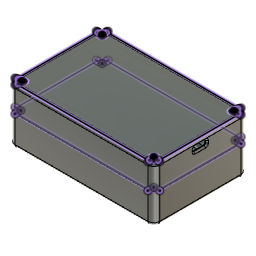
Servotester Case (Autodesk Fusion 360 design; units mm, degrees)
Autodesk Fusion 360 part; units mm, degrees
sketch "Skizze1" plane through (0, 0, 0) normal (0, 0, 1) x (1, 0, 0)
  line L0 (6.5, 58) -> (88.5, 58) construction
  line L1 (88.5, 58) -> (88.5, 21.5) construction
  line L2 (88.5, 21.5) -> (6.5, 21.5) construction
  line L3 (6.5, 21.5) -> (6.5, 58) construction
  line L4 (11.5, 52.5) -> (83.5, 52.5)
  line L5 (83.5, 52.5) -> (83.5, 27.5)
  line L6 (83.5, 27.5) -> (11.5, 27.5)
  line L7 (11.5, 27.5) -> (11.5, 52.5)
  circle A0 centre (10, 55.5) radius 1.5
  line L8 (35, 21.4) -> (61.3, 21.4) construction
  line L9 (61.3, 21.4) -> (61.3, 2.2) construction
  line L10 (61.3, 2.2) -> (35, 2.2) construction
  line L11 (35, 2.2) -> (35, 21.4) construction
  line L12 (8.4, 19.5) -> (19, 19.5) construction
  line L13 (19, 19.5) -> (19, 4.5) construction
  line L14 (19, 4.5) -> (8.4, 4.5) construction
  line L15 (8.4, 4.5) -> (8.4, 19.5) construction
  line L16 (72.4, 14.15) -> (80.4, 14.15)
  line L17 (80.4, 14.15) -> (80.4, 8.45)
  line L18 (80.4, 8.45) -> (72.4, 8.45)
  line L19 (72.4, 8.45) -> (72.4, 14.15)
  line L20 (9.25, 19.2) -> (18.15, 19.2)
  line L21 (18.15, 19.2) -> (18.15, 4.8)
  line L22 (18.15, 4.8) -> (9.25, 4.8)
  line L23 (9.25, 4.8) -> (9.25, 19.2)
  circle A1 centre (50.6, 10.1) radius 3.7
  line L24 (66.3, 21.4) -> (86.5, 21.4) construction
  line L25 (86.5, 21.4) -> (86.5, 1.2) construction
  line L26 (86.5, 1.2) -> (66.3, 1.2) construction
  line L27 (66.3, 1.2) -> (66.3, 21.4) construction
  circle A2 centre (71.32, 17.65) radius 1.5
  circle A3 centre (81.48, 17.65) radius 1.5
  circle A4 centre (71.32, 4.95) radius 1.5
  circle A5 centre (81.48, 4.95) radius 1.5
  circle A6 centre (85, 55.5) radius 1.5
  circle A7 centre (10, 24.5) radius 1.5
  circle A8 centre (85, 24.5) radius 1.5
  circle A9 centre (10, 55.5) radius 3
  circle A10 centre (85, 55.5) radius 3
  circle A11 centre (10, 24.5) radius 3
  circle A12 centre (85, 24.5) radius 3
  circle A13 centre (71.32, 17.65) radius 3
  circle A14 centre (81.48, 17.65) radius 3
  circle A15 centre (71.32, 4.95) radius 3
  circle A16 centre (81.48, 4.95) radius 3
  line L28 (2.5, 60) -> (92.5, 60)
  line L29 (95, 57.5) -> (95, 2.5)
  line L30 (92.5, 0) -> (2.5, 0)
  line L31 (0, 2.5) -> (0, 57.5)
  arc A17 (2.5, 60) -> (0, 57.5) centre (2.5, 57.5) ccw
  arc A18 (95, 57.5) -> (92.5, 60) centre (92.5, 57.5) ccw
  arc A19 (92.5, 0) -> (95, 2.5) centre (92.5, 2.5) ccw
  arc A20 (0, 2.5) -> (2.5, 0) centre (2.5, 2.5) ccw
  arc A21 (96.5, 57.5) -> (92.5, 61.5) centre (92.5, 57.5) ccw
  line L32 (2.5, 61.5) -> (92.5, 61.5)
  arc A22 (2.5, 61.5) -> (-1.5, 57.5) centre (2.5, 57.5) ccw
  line L33 (-1.5, 2.5) -> (-1.5, 57.5)
  arc A23 (-1.5, 2.5) -> (2.5, -1.5) centre (2.5, 2.5) ccw
  line L34 (92.5, -1.5) -> (2.5, -1.5)
  arc A24 (92.5, -1.5) -> (96.5, 2.5) centre (92.5, 2.5) ccw
  line L35 (96.5, 57.5) -> (96.5, 2.5)
  circle A25 centre (3, 57) radius 3
  circle A26 centre (92, 57) radius 3
  circle A27 centre (92, 3) radius 3
  circle A28 centre (3, 3) radius 3
  circle A29 centre (3, 57) radius 1.5
  circle A30 centre (92, 57) radius 1.5
  circle A31 centre (92, 3) radius 1.5
  circle A32 centre (3, 3) radius 1.5
  point P0 (0, 60)
  point P1 (95, 60)
  dimension "d3" = 82
  dimension "d4" = 36.5
  dimension "d5" = 72
  dimension "d6" = 25
  dimension "d15" = 3
  dimension "d16" = 2.5
  dimension "d20" = 26.3
  dimension "d21" = 19.2
  dimension "d22" = 10.6
  dimension "d23" = 15
  dimension "d24" = 8
  dimension "d25" = 5.7
  dimension "d26" = 8.9
  dimension "d27" = 14.4
  dimension "d28" = 0.85
  dimension "d29" = 0.3
  dimension "d30" = 7.4
  dimension "d31" = 7.9
  dimension "d32" = 10.7
  dimension "d35" = 16
  dimension "d39" = 20.2
  dimension "d40" = 20.2
  dimension "d43" = 6.1
  dimension "d44" = 7.25
  dimension "d45" = 3
  dimension "d49" = 10.16
  dimension "d50" = -12.7
  dimension "d51" = 5.02
  dimension "d52" = 3.75
  dimension "d59" = 75
  dimension "d60" = -31
  dimension "d61" = 5
  dimension "d62" = 0.1
  dimension "d63" = 0.1
  dimension "d64" = 2
  dimension "d65" = 3.5
  dimension "d66" = 2
  dimension "d67" = 6
  dimension "d68" = 5.5
  dimension "d69" = 5
  dimension "d70" = 6
  dimension "d71" = 2
  dimension "d72" = 6.5
  dimension "d74" = 60
  dimension "d75" = 2.5
  dimension "d76" = -1.5
  dimension "d83" = 6
  dimension "d84" = 6.5
  dimension "d85" = 6
  dimension "d86" = 6
  dimension "d87" = 6
  dimension "d88" = 3
  dimension "d89" = 3
  dimension "d90" = 3
  dimension "d91" = 3
  constraint horizontal L0
  constraint vertical L1
  constraint horizontal L2
  constraint vertical L3
  constraint horizontal L4
  constraint vertical L5
  constraint horizontal L6
  constraint vertical L7
  constraint horizontal L8
  constraint vertical L9
  constraint horizontal L10
  constraint vertical L11
  constraint horizontal L12
  constraint vertical L13
  constraint horizontal L14
  constraint vertical L15
  constraint horizontal L16
  constraint vertical L17
  constraint horizontal L18
  constraint vertical L19
  constraint horizontal L20
  constraint vertical L21
  constraint horizontal L22
  constraint vertical L23
  constraint horizontal L24
  constraint vertical L25
  constraint horizontal L26
  constraint vertical L27
  constraint concentric A0 A9
  constraint concentric A2 A13
  constraint horizontal L28
  constraint vertical L29
  constraint horizontal L30
  constraint vertical L31
  constraint coincident P0 L31
  constraint coincident P0 L28
  constraint tangent L31 A17
  constraint tangent L28 A17
  constraint coincident P1 L28
  constraint coincident P1 L29
  constraint tangent L28 A18
  constraint tangent L29 A18
  constraint equal A17 A18
  constraint tangent L29 A19
  constraint tangent L30 A19
  constraint equal A17 A19
  constraint coincident origin L30
  constraint coincident origin L31
  constraint tangent L30 A20
  constraint tangent L31 A20
  constraint equal A17 A20
  constraint tangent L28 A25
  constraint tangent L31 A25
  constraint tangent L28 A26
  constraint tangent L29 A26
  constraint tangent L30 A28
  constraint tangent L31 A28
  constraint tangent L30 A27
  constraint tangent L29 A27
  constraint concentric A25 A29
  constraint concentric A26 A30
  constraint concentric A27 A31
  constraint concentric A28 A32
  measures "d3" distance of L0.start L0.end
  measures "d4" distance of L0.start L2.end
  measures "d5" distance of L4.start L4.end
  measures "d6" distance of L4.start L6.end
  measures "d15" diameter of A0
  measures "d16" distance of L0 A0.centre
  measures "d20" distance of L8.start L8.end
  measures "d21" distance of L8.start L10.end
  measures "d22" distance of L12.start L12.end
  measures "d23" distance of L12.start L14.end
  measures "d24" distance of L16.start L16.end
  measures "d25" distance of L16.start L18.end
  measures "d26" distance of L20.start L20.end
  measures "d27" distance of L20.start L22.end
  measures "d28" distance of L15 L23
  measures "d29" distance of L12 L20
  measures "d30" diameter of A1
  measures "d31" distance of L10 A1.centre
  measures "d32" distance of L9 A1.centre
  measures "d35" distance of L11 L13
  measures "d39" distance of L24.start L24.end
  measures "d40" distance of L24.start L26.end
  measures "d43" distance of L19 L27
  measures "d44" distance of L18 L26
  measures "d45" diameter of A2
  measures "d51" distance of L27 A2.centre
  measures "d52" distance of L24 A2.centre
  measures "d61" distance of L9 L27
  measures "d62" distance of L2 L8
  measures "d63" distance of L2 L24
  measures "d64" distance of L2 L12
  measures "d65" distance of L3 A0.centre
  measures "d66" distance of L1 L25
  measures "d67" diameter of A9
  measures "d68" distance of L0 L4
  measures "d69" distance of L3 L7
  measures "d70" diameter of A13
  measures "d71" distance of L0 L28
  measures "d72" distance of L1 L29
  measures "d74" distance of P0 origin
  measures "d75" radius of A17
  measures "d83" diameter of A25
  measures "d84" distance of L3 L31
  measures "d85" diameter of A26
  measures "d86" diameter of A27
  measures "d87" diameter of A28
  measures "d88" diameter of A29
  measures "d89" diameter of A30
  measures "d90" diameter of A31
  measures "d91" diameter of A32
extrude "Extrusion1" add sketch "Skizze1" along normal blind 1.5 contours A0 | A2 | A3 | A4 | A5 | A6 | A7 | A8 | A9 | A10 | A11 | A12 | A13 | A14 | A15 | A16 | L28 L31 A17 A25 | L28 L29 L30 L31 A25 A26 A27 A28 | A25 | L28 L29 A18 A26 | A26 | L30 L31 A20 A28 | A28 | A27 | L29 L30 A19 A27 | A29 | A30 | A31 | A32 makes body 1
extrude "Extrusion2" add sketch "Skizze1" along normal blind 6 contours A9 | A10 | A11 | A12 bodies 1
extrude "Extrusion12" add sketch "Skizze1" along normal blind 4.4 contours A13 | A14 | A15 | A16 bodies 1
extrude "Extrusion4" add sketch "Skizze1" along normal blind 15 contours L28 L31 A17 A25 | A25 | L28 L29 A18 A26 | A26 | L30 L31 A20 A28 | A28 | A27 | L29 L30 A19 A27 bodies 1
extrude "Extrusion3" add sketch "Skizze1" along normal blind 20 contours A21 L32 A22 L33 A23 L34 A24 L35 bodies 1
fillet "Abrundung1" radius 2 8 edges at (-0.3284, -0.3284, 0) (47.5, -1.5, 0) (95.3284, -0.3284, 0) (96.5, 30, 0) (95.3284, 60.3284, 0) (47.5, 61.5, 0) (-0.3284, 60.3284, 0) (-1.5, 30, 0) on bodies 1
chamfer "Fase1" distance 0.8 angle 45 8 edges at (72.4, 11.3, 0) (80.4, 11.3, 0) (76.4, 8.45, 0) (76.4, 14.15, 0) (11.5, 40, 0) (47.5, 52.5, 0) (83.5, 40, 0) (47.5, 27.5, 0) on bodies 1
fillet "Abrundung2" radius 2 8 edges at (47.5, 0, 1.5) (95, 30, 1.5) (89.8787, 5.1213, 1.5) (5.1213, 5.1213, 1.5) (0, 30, 1.5) (5.1213, 54.8787, 1.5) (47.5, 60, 1.5) (89.8787, 54.8787, 1.5) on bodies 1
fillet "Abrundung5" radius 1 4 edges at (82.203, 25.5848, 1.5) (78.683, 18.7348, 1.5) (68.523, 18.7348, 1.5) (7.203, 25.5848, 1.5) on bodies 1
fillet "Abrundung6" radius 0.5 4 edges at (81.48, 1.95, 1.5006) (81.48, 7.95, 1.5) (71.32, 1.95, 1.5006) (71.32, 7.95, 1.5) on bodies 1
sketch "Skizze2" plane through (0, 0, 20) normal (0, 0, 1) x (-1, 0, 0)
  arc A0 (-2.5, -60) -> (0, -57.5) centre (-2.5, -57.5) ccw
  line L0 (-2.5, -60) -> (-92.5, -60)
  arc A1 (-95, -57.5) -> (-92.5, -60) centre (-92.5, -57.5) ccw
  line L1 (-95, -57.5) -> (-95, -2.5)
  arc A2 (-92.5, 0) -> (-95, -2.5) centre (-92.5, -2.5) ccw
  line L2 (-92.5, 0) -> (-2.5, 0)
  arc A3 (0, -2.5) -> (-2.5, 0) centre (-2.5, -2.5) ccw
  line L3 (0, -2.5) -> (0, -57.5)
  arc A4 (-2.5, -61.5) -> (1.5, -57.5) centre (-2.5, -57.5) ccw
  line L4 (1.5, -57.5) -> (1.5, -2.5)
  arc A5 (1.5, -2.5) -> (-2.5, 1.5) centre (-2.5, -2.5) ccw
  line L5 (-2.5, 1.5) -> (-92.5, 1.5)
  arc A6 (-92.5, 1.5) -> (-96.5, -2.5) centre (-92.5, -2.5) ccw
  line L6 (-96.5, -2.5) -> (-96.5, -57.5)
  arc A7 (-96.5, -57.5) -> (-92.5, -61.5) centre (-92.5, -57.5) ccw
  line L7 (-92.5, -61.5) -> (-2.5, -61.5)
  line L8 (-95.7, -2.5) -> (-95.7, -57.5)
  arc A8 (-95.7, -57.5) -> (-92.5, -60.7) centre (-92.5, -57.5) ccw
  line L9 (-92.5, -60.7) -> (-2.5, -60.7)
  arc A9 (-2.5, -60.7) -> (0.7, -57.5) centre (-2.5, -57.5) ccw
  line L10 (0.7, -57.5) -> (0.7, -2.5)
  arc A10 (0.7, -2.5) -> (-2.5, 0.7) centre (-2.5, -2.5) ccw
  line L11 (-2.5, 0.7) -> (-92.5, 0.7)
  arc A11 (-92.5, 0.7) -> (-95.7, -2.5) centre (-92.5, -2.5) ccw
  dimension "d99" = -0.8
extrude "Extrusion5" cut sketch "Skizze2" against normal blind 1.5 contours L8 A8 L9 A9 L10 A10 L11 A11 bodies 1
ref_plane "Arbeitsebene1" through (47.5, 30, 37) normal (0, 0, -1) x (-1, 0, 0)
sketch "Skizze3" plane through (48.2, 30, 37) normal (0, 0, -1) x (1, 0, 0)
  line L0 (47.5, -27.5) -> (47.5, 27.5)
  arc A0 (47.5, 27.5) -> (44.3, 30.7) centre (44.3, 27.5) ccw
  line L1 (44.3, 30.7) -> (-45.7, 30.7)
  arc A1 (-45.7, 30.7) -> (-48.9, 27.5) centre (-45.7, 27.5) ccw
  line L2 (-48.9, 27.5) -> (-48.9, -27.5)
  arc A2 (-48.9, -27.5) -> (-45.7, -30.7) centre (-45.7, -27.5) ccw
  line L3 (-45.7, -30.7) -> (44.3, -30.7)
  arc A3 (44.3, -30.7) -> (47.5, -27.5) centre (44.3, -27.5) ccw
  arc A4 (-49.7, -27.5) -> (-45.7, -31.5) centre (-45.7, -27.5) ccw
  line L4 (-49.7, -27.5) -> (-49.7, 27.5)
  arc A5 (-45.7, 31.5) -> (-49.7, 27.5) centre (-45.7, 27.5) ccw
  line L5 (-45.7, 31.5) -> (44.3, 31.5)
  arc A6 (48.3, 27.5) -> (44.3, 31.5) centre (44.3, 27.5) ccw
  line L6 (48.3, 27.5) -> (48.3, -27.5)
  arc A7 (44.3, -31.5) -> (48.3, -27.5) centre (44.3, -27.5) ccw
  line L7 (44.3, -31.5) -> (-45.7, -31.5)
  arc A8 (46.8, 27.5) -> (44.3, 30) centre (44.3, 27.5) ccw
  line L8 (44.3, 30) -> (-45.7, 30)
  arc A9 (-45.7, 30) -> (-48.2, 27.5) centre (-45.7, 27.5) ccw
  line L9 (-48.2, 27.5) -> (-48.2, -27.5)
  arc A10 (-48.2, -27.5) -> (-45.7, -30) centre (-45.7, -27.5) ccw
  line L10 (-45.7, -30) -> (44.3, -30)
  arc A11 (44.3, -30) -> (46.8, -27.5) centre (44.3, -27.5) ccw
  line L11 (46.8, -27.5) -> (46.8, 27.5)
  arc A12 (47.5, 27.5) -> (44.3, 30.7) centre (44.3, 27.5) ccw
  line L12 (47.5, 27.5) -> (47.5, -27.5)
  arc A13 (44.3, -30.7) -> (47.5, -27.5) centre (44.3, -27.5) ccw
  line L13 (44.3, -30.7) -> (-45.7, -30.7)
  arc A14 (-48.9, -27.5) -> (-45.7, -30.7) centre (-45.7, -27.5) ccw
  line L14 (-48.9, -27.5) -> (-48.9, 27.5)
  arc A15 (-45.7, 30.7) -> (-48.9, 27.5) centre (-45.7, 27.5) ccw
  line L15 (-45.7, 30.7) -> (44.3, 30.7)
  circle A16 centre (43.8, 27) radius 1.5
  arc A17 (46.8, 27.5) -> (44.3, 30) centre (44.3, 27.5) ccw
  line L16 (46.8, 27.5) -> (46.8, 27)
  arc A18 (43.8, 30) -> (46.8, 27) centre (43.8, 27) ccw
  line L17 (43.8, 30) -> (44.3, 30)
  circle A19 centre (-45.2, 27) radius 1.5
  arc A20 (-45.7, 30) -> (-48.2, 27.5) centre (-45.7, 27.5) ccw
  line L18 (-45.7, 30) -> (-45.2, 30)
  arc A21 (-48.2, 27) -> (-45.2, 30) centre (-45.2, 27) ccw
  line L19 (-48.2, 27) -> (-48.2, 27.5)
  circle A22 centre (-45.2, -27) radius 1.5
  arc A23 (-48.2, -27.5) -> (-45.7, -30) centre (-45.7, -27.5) ccw
  line L20 (-48.2, -27.5) -> (-48.2, -27)
  arc A24 (-45.2, -30) -> (-48.2, -27) centre (-45.2, -27) ccw
  line L21 (-45.2, -30) -> (-45.7, -30)
  circle A25 centre (43.8, -27) radius 1.5
  arc A26 (44.3, -30) -> (46.8, -27.5) centre (44.3, -27.5) ccw
  line L22 (44.3, -30) -> (43.8, -30)
  arc A27 (46.8, -27) -> (43.8, -30) centre (43.8, -27) ccw
  line L23 (46.8, -27) -> (46.8, -27.5)
  circle A28 centre (43.8, 27) radius 1.2
  circle A29 centre (43.8, 27) radius 2.1
  circle A30 centre (-45.2, 27) radius 1.2
  circle A31 centre (-45.2, 27) radius 2.1
  circle A32 centre (43.8, -27) radius 1.2
  circle A33 centre (43.8, -27) radius 2.1
  circle A34 centre (-45.2, -27) radius 1.2
  circle A35 centre (-45.2, -27) radius 2.1
  line L24 (-45.7, -30.5) -> (44.3, -30.5)
  arc A36 (44.3, -30.5) -> (47.3, -27.5) centre (44.3, -27.5) ccw
  line L25 (47.3, -27.5) -> (47.3, 27.5)
  arc A37 (47.3, 27.5) -> (44.3, 30.5) centre (44.3, 27.5) ccw
  line L26 (44.3, 30.5) -> (-45.7, 30.5)
  arc A38 (-45.7, 30.5) -> (-48.7, 27.5) centre (-45.7, 27.5) ccw
  line L27 (-48.7, 27.5) -> (-48.7, -27.5)
  arc A39 (-48.7, -27.5) -> (-45.7, -30.5) centre (-45.7, -27.5) ccw
  dimension "d111" = 2.4
  dimension "d112" = 4.2
  dimension "d113" = 2.4
  dimension "d114" = 4.2
  dimension "d115" = 2.4
  dimension "d116" = 4.2
  dimension "d117" = 2.4
  dimension "d118" = 4.2
  dimension "d126" = -0.2
  constraint concentric A16 A28
  constraint concentric A16 A29
  constraint concentric A19 A30
  constraint concentric A19 A31
  constraint concentric A25 A32
  constraint concentric A32 A33
  constraint concentric A22 A34
  constraint concentric A34 A35
  measures "d111" diameter of A28
  measures "d112" diameter of A29
  measures "d113" diameter of A30
  measures "d114" diameter of A31
  measures "d115" diameter of A32
  measures "d116" diameter of A33
  measures "d117" diameter of A34
  measures "d118" diameter of A35
extrude "Extrusion6" add sketch "Skizze3" along normal up to surface (17 mm away) separate body contours L0 A0 L1 A1 L2 A2 L3 A3 A12 L12 A13 L13 A14 L14 A15 L15 | A4 L4 A5 L5 A6 L6 A7 L7 makes body 2
extrude "Extrusion7" add sketch "Skizze3" along normal up to surface (18.5 mm away) separate body contours L24 A36 L25 A37 L26 A38 L27 A39 makes body 3
extrude "Extrusion8" add sketch "Skizze3" along normal blind 21.5 separate body contours A8 L8 L11 A17 L16 A18 L17 | L10 A11 L11 A26 L22 A27 L23 | L8 A9 L9 A20 L18 A21 L19 | L9 A10 L10 A23 L20 A24 L21 | A16 | A19 | A22 | A25 | A29 | A31 | A33 | A35 makes body 4 at (93.7871, 54.5904, 22.6667) makes body 5 at (0.0036, 56.8528, 22.6667) makes body 6 at (90.9893, 0.1754, 22.6667) makes body 7 at (3.2941, 0.0144, 22.6667)
combine "Kombinieren1" operation add target body 3 tool bodies 4 5 2 6 7
extrude "Extrusion9" add sketch "Skizze3" along normal blind 1.5 contours L0 A0 L1 A1 L2 A2 L3 A3 A12 L12 A13 L13 A14 L14 A15 L15 | A4 L4 A5 L5 A6 L6 A7 L7 | A8 L8 L11 A17 L16 A18 L17 | L8 L9 L10 L11 A18 A21 A24 A27 | L10 A11 L11 A26 L22 A27 L23 | L8 A9 L9 A20 L18 A21 L19 | L9 A10 L10 A23 L20 A24 L21 | A16 | A19 | A22 | A25 | A29 | A31 | A33 | A35 | L24 A36 L25 A37 L26 A38 L27 A39 bodies 3
extrude "Extrusion10" cut sketch "Skizze3" along normal blind 17 contours A16 | A19 | A22 | A25 | A29 | A31 | A33 | A35 bodies 3
chamfer "Fase2" distance 0.9 angle 45 4 edges at (90.8812, 2.5661, 20) (90.8812, 56.5661, 20) (1.8812, 2.5661, 20) (1.8812, 56.5661, 20) on bodies 3
fillet "Abrundung3" radius 2 8 edges at (95.3284, -0.3284, 37) (47.5, -1.5, 37) (-0.3284, -0.3284, 37) (-1.5, 30, 37) (-0.3284, 60.3284, 37) (47.5, 61.5, 37) (95.3284, 60.3284, 37) (96.5, 30, 37) on bodies 3
fillet "Abrundung4" radius 2 7 edges at (47.5, 60, 35.5) (89.8787, 54.8787, 35.5) (47.5, 0, 35.5) (89.8787, 5.1213, 35.5) (5.1213, 5.1213, 35.5) (0, 30, 35.5) (5.1213, 54.8787, 35.5) on bodies 3
sketch "Skizze5" plane through (96.5, 0, 0) normal (1, 0, 0) x (0, 1, 0)
  line L0 (57.5, 35) -> (2.5, 35)
  line L1 (2.5, 35) -> (2.5, 20)
  line L2 (2.5, 20) -> (57.5, 20)
  line L3 (57.5, 20) -> (57.5, 35)
  line L4 (57.5, 37) -> (2.5, 37)
  line L5 (2.5, 35) -> (57.5, 35)
  line L6 (2.5, 35) -> (-1.5, 35)
  line L7 (-1.5, 35) -> (-1.5, 20)
  line L8 (-1.5, 20) -> (2.5, 20)
  line L9 (2.5, 20) -> (2.5, 35)
  line L10 (61.5, 35) -> (57.5, 35)
  line L11 (57.5, 35) -> (57.5, 20)
  line L12 (57.5, 20) -> (61.5, 20)
  line L13 (61.5, 20) -> (61.5, 35)
  line L14 (61.5, 35) -> (57.5, 35)
  line L15 (2.5, 35) -> (-1.5, 35)
  line L16 (26.5, 33.9) -> (33.5, 33.9)
  line L17 (34.5, 32.9) -> (34.5, 31.5)
  line L18 (33.5, 30.5) -> (26.5, 30.5)
  line L19 (25.5, 31.5) -> (25.5, 32.9)
  arc A0 (26.5, 33.9) -> (25.5, 32.9) centre (26.5, 32.9) ccw
  arc A1 (25.5, 31.5) -> (26.5, 30.5) centre (26.5, 31.5) ccw
  arc A2 (33.5, 30.5) -> (34.5, 31.5) centre (33.5, 31.5) ccw
  arc A3 (34.5, 32.9) -> (33.5, 33.9) centre (33.5, 32.9) ccw
  line L20 (57.5, 35) -> (57.5, 37)
  line L21 (2.5, 37) -> (2.5, 35)
  line L22 (57.5, 35) -> (57.5, 37)
  arc A4 (61.5, 35) -> (59.5, 37) centre (59.5, 35) ccw
  line L23 (57.5, 37) -> (59.5, 37)
  line L24 (2.5, 37) -> (2.5, 35)
  line L25 (0.5, 37) -> (2.5, 37)
  arc A5 (0.5, 37) -> (-1.5, 35) centre (0.5, 35) ccw
  point P0 (25.5, 33.9)
  point P1 (34.5, 33.9)
  point P2 (25.5, 30.5)
  point P3 (30, 33.9)
  dimension "d132" = 9
  dimension "d133" = 3.4
  dimension "d134" = 1
  dimension "d135" = 55
  dimension "d136" = 27.5
  dimension "d137" = 3.1
  constraint horizontal L16
  constraint vertical L17
  constraint horizontal L18
  constraint vertical L19
  constraint coincident P0 L16
  constraint coincident P0 L19
  constraint tangent L16 A0
  constraint tangent L19 A0
  constraint coincident P2 L19
  constraint coincident P2 L18
  constraint tangent L19 A1
  constraint tangent L18 A1
  constraint equal A0 A1
  constraint tangent L17 A2
  constraint tangent L18 A2
  constraint equal A0 A2
  constraint coincident P1 L16
  constraint coincident P1 L17
  constraint tangent L16 A3
  constraint tangent L17 A3
  constraint equal A0 A3
  constraint midpoint L16 P3
  measures "d132" distance of P0 P1
  measures "d133" distance of P0 P2
  measures "d134" radius of A0
  measures "d135" distance of L0.start L0.end
  measures "d136" distance of L1 P3
  measures "d137" distance of L4 L16
extrude "Extrusion11" cut sketch "Skizze5" against normal blind 1.5 contours L16 L17 L18 L19 A0 A1 A2 A3 bodies 3
chamfer "Fase3" distance 1 angle 45 8 edges at (96.5, 30, 33.9) (96.5, 34.2071, 33.6071) (96.5, 34.5, 32.2) (96.5, 34.2071, 30.7929) (96.5, 30, 30.5) (96.5, 25.7929, 30.7929) (96.5, 25.5, 32.2) (96.5, 25.7929, 33.6071) on bodies 3
equation "d28 = ( d22 - d26 ) / 2"
equation "d29 = ( d23 - d27 ) / 2"
equation "d43 = ( d39 - d24 ) / 2"
equation "d44 = ( d40 - d25 ) / 2"
equation "d51 = ( d39 - 10.16 mm ) / 2"
equation "d52 = ( d39 - 12.7 mm ) / 2"
equation "d136 = d135 / 2"
named bodies: "Servotester Case Top", "Servotester Case Bottom"
